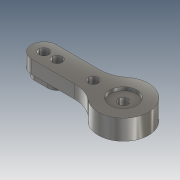
# Autodesk Inventor part: servo-metal-arm
Saved by Autodesk Inventor 2017 (Build 210142000, 142)
## iProperties
Created: 2018-05-01
Part Number: servo-metal-arm
Material: Generic
Document SubType Name: Modeling
Designer: Luiz Gustavo
Density: 1 g/cm^3
Appearance: Chrome - Polished
Author: Luiz Gustavo
Autodesk Inventor part; units mm, degrees
ref_plane "YZ Plane" through (0, 0, 0) normal (1, 0, 0) x (0, 1, 0)
ref_plane "XZ Plane" through (0, 0, 0) normal (0, 1, 0) x (-1, 0, 0)
ref_plane "XY Plane" through (0, 0, 0) normal (0, 0, 1) x (1, 0, 0)
sketch "Sketch2" plane through (0, 0, 0) normal (0, 0, 1) x (1, 0, 0)
  circle A0 centre (0, 0) radius 1.5
  circle A1 centre (0, 0) radius 4
  arc A2 (-6.5238, 3.7) -> (-6.5238, -3.7) centre (0, 0) ccw construction
  line L0 (7.5, 0) -> (-27.5, 0) construction
  arc A3 (-23.8, -3.7) -> (-23.8, 3.7) centre (-23.8, 0) ccw construction
  circle A4 centre (-23.8, 0) radius 1.5
  circle A5 centre (-19.8, 0) radius 1.5
  line L1 (-23.8, 3.7) -> (-10.8885, 3.7)
  line L2 (-23.8, -3.7) -> (-10.8885, -3.7)
  arc A6 (-27.5, 0) -> (-23.8, -3.7) centre (-23.8, 0) ccw
  arc A7 (-23.8, 3.7) -> (-27.5, 0) centre (-23.8, 0) ccw
  arc A8 (7.5, 0) -> (-4.6665, 5.8714) centre (0, 0) ccw
  arc A9 (-6.5238, -3.7) -> (-4.6665, -5.8714) centre (0, 0) ccw construction
  circle A10 centre (-9, 0) radius 1.5
  arc A11 (-10.8885, 3.7) -> (-4.6665, 5.8714) centre (-10.8885, 13.7) ccw
  arc A12 (-4.6665, -5.8714) -> (-10.8885, -3.7) centre (-10.8885, -13.7) ccw
  arc A13 (-4.6665, -5.8714) -> (7.5, 0) centre (0, 0) ccw
  line L3 (-10.8885, -13.7) -> (-10.8885, 13.7) construction
  line L4 (-23.8, 0) -> (-19.8, 0) construction
  line L5 (-23.8, -2.85) -> (-19.8, -2.85)
  line L6 (-19.8, 2.85) -> (-23.8, 2.85)
  arc A14 (-23.8, 2.85) -> (-23.8, -2.85) centre (-23.8, 0) ccw
  arc A15 (-19.8, -2.85) -> (-19.8, 2.85) centre (-19.8, 0) ccw
  arc A16 (-4.6665, 5.8714) -> (-4.6665, -5.8714) centre (0, 0) ccw
  point P0 (-21.8, 0)
  dimension "d12" = 35
  dimension "d13" = 15
  dimension "d14" = 7.4
  dimension "d15" = 3
  dimension "d16" = 8
  dimension "d17" = 3
  dimension "d18" = 4
  dimension "d19" = 9
  dimension "d20" = 10
  dimension "d21" = 2.85
  constraints: 24 point on circle, 17 centre point, 16 end point, 12 tangent, 5 coincident, 4 point on line, 3 equal radius, 3 horizontal, 1 collinear, 1 midpoint, 1 parallel, 1 vertical
  measures "d12" distance of L0.start L0.end
  measures "d13" diameter of A2
  measures "d14" diameter of A3
  measures "d15" diameter of A0
  measures "d16" diameter of A1
  measures "d17" diameter of A4
  measures "d18" distance of A3.centre L4.end
  measures "d19" distance of A10.centre point (0, 0)
  measures "d20" radius of A11
  measures "d21" radius of A15
extrude "Extrusion3" add sketch "Sketch2" along normal blind 4 contours L1 A11 A16 A12 L2 A6 A7 | A8 A13 A16 | A14 L6 A15 L5
extrude "Extrusion4" add sketch "Sketch2" along normal blind 3 contours A1
extrude "Extrusion5" add sketch "Sketch2" against normal blind 2 contours A8 A13 A16 | A14 L6 A15 L5
body "Solid2"
